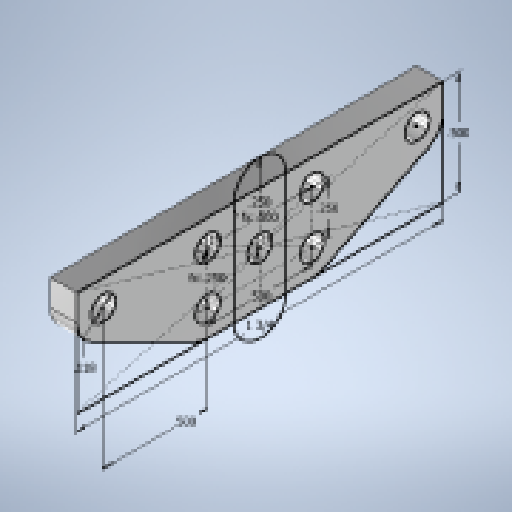
# Autodesk Inventor part: Pin Cap
Saved by Autodesk Inventor 2023.2 (Build 272271000, 271)
## iProperties
Created: 2024-02-03
Part Number: Pin Cap
Material: Aluminum 6061
Document SubType Name: Modeling
Designer: Nathan Cai
Density: 2.7 g/cm^3
Appearance: Aluminum - Flat
Mass: 2.66009 g
Surface Area: 11.284 cm^2
Volume: 0.985219 cm^3
Author: Nathan Cai
Autodesk Inventor part; units mm, degrees
ref_plane "YZ Plane" through (0, 0, 0) normal (1, 0, 0) x (0, 1, 0)
ref_plane "XZ Plane" through (0, 0, 0) normal (0, 1, 0) x (-1, 0, 0)
ref_plane "XY Plane" through (0, 0, 0) normal (0, 0, 1) x (1, 0, 0)
sketch "Sketch1" plane through (0, 0, 0) normal (1, 0, 0) x (0, 1, 0)
  line L0 (3.175, 6.35) -> (-3.175, 6.35) construction
  line L1 (-3.175, 6.35) -> (-3.175, -6.35) construction
  line L2 (-3.175, -6.35) -> (3.175, -6.35) construction
  line L3 (3.175, -6.35) -> (3.175, 6.35) construction
  line L4 (3.175, 6.35) -> (-3.175, -6.35) construction
  line L5 (-3.175, 6.35) -> (3.175, -6.35) construction
  circle A0 centre (0, 0) radius 1.5
  circle A1 centre (3.175, 6.35) radius 1.5
  circle A2 centre (3.175, -6.35) radius 1.5
  circle A3 centre (-3.175, 6.35) radius 1.5
  circle A4 centre (-3.175, -6.35) radius 1.5
  line L6 (6.35, 22.225) -> (-6.35, 22.225)
  line L7 (-6.35, 22.225) -> (-6.35, -22.225)
  line L8 (-6.35, -22.225) -> (6.35, -22.225)
  line L9 (6.35, -22.225) -> (6.35, 22.225)
  line L10 (6.35, 22.225) -> (-6.35, -22.225) construction
  line L11 (-6.35, 22.225) -> (6.35, -22.225) construction
  line L12 (-6.35, 0) -> (6.35, 0) construction
  line L13 (-6.35, -3.175) -> (6.35, -3.175)
  line L14 (6.35, 3.175) -> (-6.35, 3.175)
  arc A5 (-6.35, 3.175) -> (-6.35, -3.175) centre (-6.35, 0) ccw
  arc A6 (6.35, -3.175) -> (6.35, 3.175) centre (6.35, 0) ccw
  circle A7 centre (3.175, 19.05) radius 1.5
  arc A8 (3.175, 22.225) -> (0.3352, 20.4699) centre (3.175, 19.05) ccw
  arc A9 (-6.0148, 7.7699) -> (-6.35, 6.35) centre (-3.175, 6.35) ccw
  line L15 (0.3352, 20.4699) -> (-6.0148, 7.7699)
  circle A10 centre (3.175, -19.05) radius 1.5
  arc A11 (0.3352, -20.4699) -> (3.175, -22.225) centre (3.175, -19.05) ccw
  arc A12 (-6.35, -6.35) -> (-6.0148, -7.7699) centre (-3.175, -6.35) ccw
  line L16 (0.3352, -20.4699) -> (-6.0148, -7.7699)
  point P0 (3.175, -22.225)
  point P1 (-6.35, -6.35)
  dimension "d0" = 6.35
  dimension "d1" = 12.7
  dimension "d2" = 3
  dimension "d3" = 3
  dimension "d6" = 12.7
  dimension "d9" = 6.35
  dimension "d12" = 12.7
  dimension "d13" = 44.45
  dimension "d14" = 6.35
  dimension "d20" = 3
  dimension "d21" = 12.7
  constraints: 36 end point, 13 centre point, 12 point on circle, 8 tangent, 7 symmetric about line, 6 midpoint, 5 coincident, 5 parallel, 3 horizontal, 3 point on line, 2 perpendicular, 1 vertical, 9 other
  measures "d0" distance of L2.end L1.end
  measures "d1" distance of L1.end L0.end
  measures "d2" diameter of A0
  measures "d3" diameter of A1
  measures "d6" distance of A1.centre A2.centre
  measures "d9" distance of A1.centre A3.centre
  measures "d12" distance of L8.end L7.end
  measures "d13" distance of L7.end L6.end
  measures "d14" diameter of A6
  measures "d20" diameter of A7
  measures "d21" distance of A1.centre A7.centre
extrude "Extrusion2" add sketch "Sketch1" against normal blind 3.175 contours L9 L14 L7 A9 L15 A8 L6 | L9 L13 L7 L14 | L9 L8 A11 L16 A12 L7 L13
equation "\"d6\" = d1"
equation "\"d9\" = d0"
body "Solid1"
